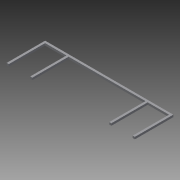
# Autodesk Inventor part: banner holder
Saved by Autodesk Inventor 2014 (Build 180170000, 170)
## iProperties
Created: 2015-04-10
Part Number: banner holder
Material: Generic
Document SubType Name: Modeling
Designer: Gus
Density: 1 g/cm^3
Appearance: Default
Author: Gus
Autodesk Inventor part; units mm, degrees
ref_plane "YZ Plane" through (0, 0, 0) normal (1, 0, 0) x (0, 1, 0)
ref_plane "XZ Plane" through (0, 0, 0) normal (0, 1, 0) x (-1, 0, 0)
ref_plane "XY Plane" through (0, 0, 0) normal (0, 0, 1) x (1, 0, 0)
sketch "Sketch1" plane through (0, 0, 0) normal (0, 1, 0) x (-1, 0, 0)
  line L0 (0, 0) -> (3048, 0)
  line L1 (3048, 0) -> (3048, 914.4)
  line L2 (3048, 914.4) -> (0, 914.4)
  line L3 (0, 914.4) -> (0, 0)
  dimension "d0" = 3048
  dimension "d1" = 914.4
  constraints: 8 end point, 2 parallel, 1 horizontal, 1 perpendicular
  measures "d0" distance of L2.end L1.end
  measures "d1" distance of L1.end L0.end
extrude "Extrusion1" add sketch "Sketch1" along normal blind 50.8
sketch "Sketch2" plane through (0, 50.8, 0) normal (0, 1, 0) x (1, 0, 0)
  line L0 (-3048, -914.4) -> (0, -914.4) projected
  line L1 (-2997.2, -914.4) -> (-50.8, -914.4)
  line L2 (-50.8, -914.4) -> (-50.8, -50.8)
  line L3 (-50.8, -50.8) -> (-2997.2, -50.8)
  line L4 (-2997.2, -50.8) -> (-2997.2, -914.4)
  dimension "d4" = 2946.4
  dimension "d5" = 863.6
  constraints: 8 end point, 2 parallel, 1 horizontal, 1 perpendicular, 1 point on line
  measures "d4" distance of L3.end L2.end
  measures "d5" distance of L2.end L1.end
extrude "Extrusion2" cut sketch "Sketch2" against normal blind 442.9125
sketch "Sketch3" plane through (0, 50.8, 0) normal (0, 1, 0) x (1, 0, 0)
  line L0 (-50.8, -50.8) -> (-50.8, -914.4) projected
  line L1 (-2997.2, -914.4) -> (-2997.2, -50.8) projected
  line L2 (-2997.2, -50.8) -> (-50.8, -50.8) projected
  line L3 (-558.8, -50.8) -> (-609.6, -50.8)
  line L4 (-609.6, -50.8) -> (-609.6, -914.4)
  line L5 (-609.6, -914.4) -> (-558.8, -914.4)
  line L6 (-558.8, -914.4) -> (-558.8, -50.8)
  line L7 (-2489.2, -50.8) -> (-2438.4, -50.8)
  line L8 (-2438.4, -50.8) -> (-2438.4, -914.4)
  line L9 (-2438.4, -914.4) -> (-2489.2, -914.4)
  line L10 (-2489.2, -914.4) -> (-2489.2, -50.8)
  dimension "d8" = 50.8
  dimension "d9" = 50.8
  dimension "d10" = 508
  dimension "d11" = 508
  constraints: 16 end point, 4 parallel, 2 horizontal, 2 perpendicular, 2 point on line
  measures "d8" distance of L5.end L4.end
  measures "d9" distance of L8.end L9.end
  measures "d10" distance between parallel lines of L10 L1
  measures "d11" distance between parallel lines of L0 L6
extrude "Extrusion3" add sketch "Sketch3" against normal blind 50.8
body "Solid1"
